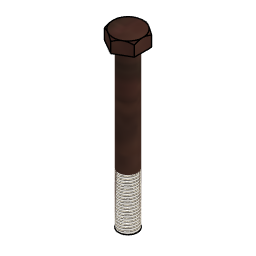
assignment1d-hexscrew (Autodesk Fusion 360 design; units mm, degrees)
Autodesk Fusion 360 part; units mm, degrees
sketch "Sketch1" plane through (0, 0, 0) normal (0, 0, 1) x (1, 0, 0) in component "Hex screw"
  circle A0 centre (0, 0) radius 6.25
  dimension "d1" = 12.5
  constraint coincident A0.centre origin
  measures "d1" diameter of A0
extrude "Extrude1" add sketch "Sketch1" along normal blind 108 in component "Hex screw"
thread "Thread1" "ISO Metric profile 12.0 M12x1.75 6g" major diameter 11.8335 minor diameter 9.8365 pitch 1.75 angle 60 resizes the face on face at (6.2422, -0.3115, 72) from (0, 0, 0) to (0, 0, 32.5) in component "Hex screw"
sketch "Sketch2" plane through (0, 0, 108) normal (0, 0, 1) x (-1, 0, 0) in component "Hex screw"
  circle A0 centre (0, 0) radius 5.9167
  line L0 (-9.4, -5.4271) -> (0, -10.8542)
  line L1 (0, -10.8542) -> (9.4, -5.4271)
  line L2 (9.4, -5.4271) -> (9.4, 5.4271)
  line L3 (9.4, 5.4271) -> (0, 10.8542)
  line L4 (0, 10.8542) -> (-9.4, 5.4271)
  line L5 (-9.4, 5.4271) -> (-9.4, -5.4271)
  dimension "d6" = 18.8
  constraint coincident A0.centre origin
  constraint vertical L2
  measures "d6" distance of L2 L5
extrude "Extrude2" add sketch "Sketch2" against normal blind 8 in component "Hex screw"
sketch "Sketch3" plane through (0, 0, 108) normal (0, 0, 1) x (-1, 0, 0) in component "Hex screw"
  line L0 (-9.4, 5.4271) -> (-9.4, -5.4271)
  line L1 (-9.4, -5.4271) -> (0, -10.8542)
  line L2 (0, -10.8542) -> (9.4, -5.4271)
  line L3 (9.4, -5.4271) -> (9.4, 5.4271)
  line L4 (9.4, 5.4271) -> (0, 10.8542)
  line L5 (0, 10.8542) -> (-9.4, 5.4271)
  circle A0 centre (0, 0) radius 9.4
  constraint coincident A0.centre origin
  constraint tangent L0 A0
delete_face "DeleteFace1" 1 faces at (5.8873, 0.5891, 66.6667) in component "Hex screw"
extrude "Extrude3" cut sketch "Sketch3" against normal blind 8 draft 45 contours A0 keep common part in component "Hex screw"
sketch "Sketch4" plane through (0, 0, 100) normal (0, 0, -1) x (1, 0, 0) in component "Hex screw"
  line L0 (9.4, -5.4271) -> (9.4, 5.4271)
  line L1 (9.4, 5.4271) -> (0, 10.8542)
  line L2 (0, 10.8542) -> (-9.4, 5.4271)
  line L3 (-9.4, 5.4271) -> (-9.4, -5.4271)
  line L4 (-9.4, -5.4271) -> (0, -10.8542)
  line L5 (0, -10.8542) -> (9.4, -5.4271)
  circle A0 centre (0, 0) radius 6.25
  dimension "d11" = 12.5
  constraint coincident A0.centre origin
  measures "d11" diameter of A0
extrude "Extrude4" add sketch "Sketch4" along normal blind 100 contours A0 in component "Hex screw"
thread "Thread2" "ISO Metric profile 12.0 M12x1.75 6g" major diameter 11.8335 minor diameter 9.8365 pitch 1.75 angle 60 resizes the face on face at (6.2189, 0.6223, 66.6667) from (0, 0, 32.5) to (0, 0, 0) in component "Hex screw"
component "Hex screw" placed x (1, 0, 0) y (0, 1, 0) z (0, 0, 1) at (0, 0, 0)
